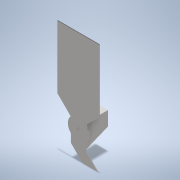
# Autodesk Inventor part: rightside0
Saved by Autodesk Inventor 2020 (Build 240168000, 168)
## iProperties
Created: 2020-04-30
Part Number: rightside0
Material: Generic
Document SubType Name: Modeling
Designer: LENOVO
Density: 1 g/cm^3
Appearance: Default
Author: LENOVO
Autodesk Inventor part; units mm, degrees
sketch "Sketch1" plane through (0, 0, 0) normal (0, 0, 1) x (1, 0, 0)
  line L0 (-100, 150) -> (100, 150)
  line L1 (100, 150) -> (100, -150)
  line L2 (-100, -150) -> (-100, 150)
  line L3 (-100, 150) -> (100, -150) construction
  line L4 (100, 150) -> (-100, -150) construction
  line L5 (100, -150) -> (36.4382, -213.5618)
  line L6 (-35.3571, -283.1536) -> (-35.3571, -323.1554)
  line L7 (-35.3571, -323.1554) -> (21.2114, -379.7239)
  line L8 (35.3571, -283.1536) -> (35.3571, -323.1554)
  line L9 (35.3571, -323.1554) -> (91.9257, -379.7239)
  line L10 (91.9257, -379.7239) -> (21.2114, -379.7239)
  arc A0 (-35.3571, -283.1536) -> (-35.3553, -283.1554) centre (0, -247.8) ccw
  arc A1 (-36.4382, -213.5618) -> (-35.3553, -283.1554) centre (0, -247.8) ccw
  arc A2 (35.3571, -283.1536) -> (36.4382, -213.5618) centre (0, -247.8) ccw
  line L11 (-100, -150) -> (-36.4382, -213.5618)
  point P0 (0, 0)
  point P1 (35.3571, -285.3571)
  constraints: 24 end point, 7 point on circle, 3 centre point, 2 horizontal, 2 midpoint, 1 parallel, 1 perpendicular, 1 point on line, 1 vertical
extrude "Extrusion1" add sketch "Sketch1" along normal blind 3
sketch "Sketch3" plane through (0, 0, 0) normal (0, 0, -1) x (-1, 0, 0)
  arc A0 (-36.4382, -213.5618) -> (-35.3571, -283.1536) centre (0, -247.8) ccw projected
  circle A1 centre (0, -247.8) radius 2.5
  circle A2 centre (0, -247.8) radius 4.75
  circle A3 centre (0, -247.8) radius 7.5
  point P0 (0, 0)
  dimension "d27" = 5
  dimension "d28" = 9.5
  dimension "d29" = 15
  constraints: 3 centre point, 3 coincident
  measures "d27" diameter of A1
  measures "d28" diameter of A2
  measures "d29" diameter of A3
extrude "Extrusion4" cut sketch "Sketch3" against normal blind 3 contours A1
extrude "Extrusion5" add sketch "Sketch3" along normal blind 2 contours A3
sketch "Sketch4" plane through (0, 0, 0) normal (0, 0, -1) x (-1, 0, 0)
  line L0 (-30, -275.6) -> (30, -275.6)
  line L1 (30, -275.6) -> (30, -278.6)
  line L2 (30, -278.6) -> (-30, -278.6)
  line L3 (-30, -278.6) -> (-30, -275.6)
  line L4 (-30, -275.6) -> (30, -278.6) construction
  line L5 (30, -275.6) -> (-30, -278.6) construction
  circle A0 centre (0, -247.8) radius 2.5 projected
  point P0 (0, 0)
  point P1 (0, -277.1)
  dimension "d34" = 60
  dimension "d35" = 3
  dimension "d36" = 27.8
  constraints: 12 end point, 2 midpoint, 2 parallel, 1 horizontal, 1 perpendicular
  measures "d34" distance of L1.end L2.end
  measures "d35" distance of L0.end L1.end
  measures "d36" distance from line of A0.centre L0
extrude "Extrusion6" add sketch "Sketch4" along normal blind 108.75 contours L0 L1 L2 L3
ref_plane "Work Plane1" through (30, -275.6, -108.75) normal (1, 0, 0) x (0, 0, -1)
sketch "Sketch5" plane through (30, -275.6, -108.75) normal (1, 0, 0) x (0, 0, -1)
  line L0 (-108.75, 62.0382) -> (-108.75, -7.5536) projected
  line L1 (0, 0) -> (141.4214, 0) construction
  line L2 (-108.75, -47.5554) -> (-111.75, -47.5554) projected
  line L3 (-108.75, -3) -> (0, -3) projected
  line L4 (-108.75, -47.5554) -> (0, -3)
  line L5 (0, -3) -> (-108.75, -3)
  line L6 (-108.75, -3) -> (-108.75, -47.5554)
  point P0 (-108.75, 275.6)
  point P1 (-108.75, 0)
  point P2 (-108.75, 100)
  constraints: 8 end point, 1 collinear, 1 horizontal, 1 perpendicular, 1 point on line
ref_plane "Work Plane2" through (0, -278.6, 0) normal (1, 0, 0) x (0, 0, -1)
extrude "Extrusion8" add sketch "Sketch5" against normal blind 3
ref_plane "Work Plane3" through (0, -275.6, 0) normal (1, 0, 0) x (0, 0, -1)
mirror "Mirror2" about plane through (0, -275.6, 0) normal (1, 0, 0) of "Extrusion8"
sketch "Sketch6" plane through (0, 0, 0) normal (0, 0, -1) x (-1, 0, 0)
  line L0 (-15, -219.8) -> (15, -219.8)
  line L1 (15, -219.8) -> (15, -222.8)
  line L2 (15, -222.8) -> (-15, -222.8)
  line L3 (-15, -222.8) -> (-15, -219.8)
  line L4 (-15, -219.8) -> (15, -222.8) construction
  line L5 (15, -219.8) -> (-15, -222.8) construction
  circle A0 centre (0, -247.8) radius 2.5 projected
  point P0 (0, 0)
  point P1 (0, -221.3)
  dimension "d46" = 30
  dimension "d47" = 3
  dimension "d48" = 25
  constraints: 12 end point, 2 midpoint, 2 parallel, 1 horizontal, 1 perpendicular
  measures "d46" distance of L1.end L2.end
  measures "d47" distance of L0.end L1.end
  measures "d48" distance from line of L2 A0.centre
extrude "Extrusion9" add sketch "Sketch6" along normal blind 40 contours L0 L1 L2 L3
sketch "Sketch7" plane through (-15, -219.8, 0) normal (0, 1, 0) x (1, 0, 0)
  circle A0 centre (15, 2.7) radius 1.5
  line L0 (115, 0) -> (-85, 0) projected
  line L1 (19, 6.2) -> (11, 6.2)
  line L2 (11, 6.2) -> (11, 18.2)
  line L3 (11, 18.2) -> (19, 18.2)
  line L4 (19, 18.2) -> (19, 6.2)
  line L5 (19, 6.2) -> (11, 18.2) construction
  line L6 (11, 6.2) -> (19, 18.2) construction
  circle A1 centre (15, 21.7) radius 1.5
  line L7 (21.5, 25.2) -> (0, 25.2)
  line L8 (1, 33.2) -> (21.5, 33.2)
  line L9 (21.5, 33.2) -> (21.5, 25.2)
  line L10 (21.5, 25.2) -> (8.5, 33.2) construction
  line L11 (8.5, 25.2) -> (21.5, 33.2) construction
  line L12 (1, 33.2) -> (0, 33.2)
  line L13 (0, 0) -> (0, 40) projected
  point P0 (15, 0)
  point P1 (15, 12.2)
  point P2 (15, 29.2)
  dimension "d51" = 3
  dimension "d52" = 2.7
  dimension "d53" = 8
  dimension "d54" = 12
  dimension "d55" = 3.5
  dimension "d56" = 3
  dimension "d57" = 3.5
  dimension "d60" = 3.5
  constraints: 24 end point, 5 point on line, 4 midpoint, 3 horizontal, 3 parallel, 2 centre point, 1 perpendicular
  measures "d51" diameter of A0
  measures "d52" distance from line of L0 A0.centre
  measures "d53" distance of L2.end L3.end
  measures "d54" distance of L1.end L2.end
  measures "d55" distance from line of A0.centre L1
  measures "d56" diameter of A1
  measures "d57" distance from line of L3 A1.centre
  measures "d60" distance from line of A1.centre L7
extrude "Extrusion10" cut sketch "Sketch7" against normal mid plane 10
sketch "Sketch8" plane through (-30, -275.6, 0) normal (0, 1, 0) x (1, 0, 0)
  line L0 (0, 0) -> (0, 108.75)
  line L1 (0, 108.75) -> (60, 108.75)
  line L2 (60, 108.75) -> (60, 0)
  line L3 (60, 0) -> (0, 108.75) construction
  line L4 (0, 0) -> (60, 108.75) construction
  line L5 (57, 105.75) -> (3, 105.75)
  line L6 (3, 105.75) -> (3, 0)
  line L7 (57, 0) -> (57, 105.75)
  line L8 (60, 0) -> (57, 0)
  line L9 (3, 0) -> (0, 0)
  point P0 (30, 0)
  point P1 (30, 54.375)
  constraints: 20 end point, 4 parallel, 2 horizontal, 2 midpoint, 2 perpendicular
extrude "Extrusion11" add sketch "Sketch8" along normal blind 62
sketch "Sketch9" plane through (-30, -213.6, 0) normal (0, 1, 0) x (1, 0, 0)
  line L0 (0, 0) -> (0, 108.75) projected
  line L1 (60, 0) -> (0, 0)
  line L2 (0, 0) -> (0, 108.75)
  line L3 (0, 108.75) -> (60, 108.75)
  line L4 (60, 108.75) -> (60, 0)
  point P0 (30, 0)
  constraints: 8 end point, 2 parallel, 1 horizontal, 1 perpendicular
extrude "Extrusion12" add sketch "Sketch9" along normal blind 3
body "Solid1"
